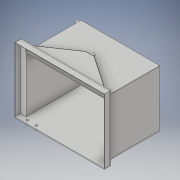
# Autodesk Inventor part: Tank2
Saved by Autodesk Inventor 2019 (Build 230136000, 136)
## iProperties
Created: 2020-03-11
Part Number: Tank2
Material: Generic
Document SubType Name: Modeling
Designer: Vijay
Density: 1 g/cm^3
Appearance: Default
Author: Vijay
Autodesk Inventor part; units mm, degrees
ref_plane "YZ Plane" through (0, 0, 0) normal (1, 0, 0) x (0, 1, 0)
ref_plane "XZ Plane" through (0, 0, 0) normal (0, 1, 0) x (-1, 0, 0)
ref_plane "XY Plane" through (0, 0, 0) normal (0, 0, 1) x (1, 0, 0)
sketch "Sketch1" plane through (0, 0, 0) normal (0, 0, 1) x (1, 0, 0)
  line L0 (-204, -167.1829) -> (204, -167.1829) construction
  line L1 (204, -167.1829) -> (204, 115) construction
  line L2 (204, 115) -> (-204, 115) construction
  line L3 (-204, 115) -> (-204, -167.1829) construction
  line L4 (-214, -177.1829) -> (214, -177.1829)
  line L5 (214, -177.1829) -> (214, 125)
  line L6 (214, 125) -> (-214, 125)
  line L7 (-214, 125) -> (-214, -177.1829)
  line L8 (-244, -177.1829) -> (244, -177.1829)
  line L9 (244, -177.1829) -> (244, 175)
  line L10 (244, 175) -> (-244, 175)
  line L11 (-244, 175) -> (-244, -177.1829)
  point P0 (0, 0)
  dimension "d0" = 10
  dimension "d1" = 30
  dimension "d2" = 30
  dimension "d3" = 50
  constraints: 24 end point, 6 parallel, 3 perpendicular, 2 horizontal, 5 other
  measures "d0" distance between parallel lines of L3 L7
  measures "d1" distance between parallel lines of L7 L11
  measures "d2" distance between parallel lines of L9 L5
  measures "d3" distance between parallel lines of L6 L10
extrude "Extrusion1" add sketch "Sketch1" along normal blind 5 contours L8 L11 L10 L9 L5 L6 L7
sketch "Sketch2" plane through (0, 0, 5) normal (0, 0, 1) x (1, 0, 0)
  line L0 (-214, -177.1829) -> (-214, 125) projected
  line L1 (-214, 125) -> (214, 125) projected
  line L2 (214, 125) -> (214, -177.1829) projected
  line L3 (214, -177.1829) -> (244, -177.1829) projected
  line L4 (244, -177.1829) -> (244, 175) projected
  line L5 (244, 175) -> (-244, 175) projected
  line L6 (-244, 175) -> (-244, -177.1829) projected
  line L7 (-244, -177.1829) -> (-214, -177.1829) projected
  line L8 (213.2, 124.2) -> (-213.2, 124.2)
  line L9 (-213.2, 124.2) -> (-213.2, -176.3829)
  line L10 (-244, -177.9829) -> (-244.8, -177.9829)
  line L11 (-244.8, -177.9829) -> (-244.8, 175.8)
  line L12 (-244.8, 175.8) -> (244.8, 175.8)
  line L13 (244.8, 175.8) -> (244.8, -177.9829)
  line L14 (244.8, -177.9829) -> (213.2, -177.9829)
  line L15 (214, 125) -> (214, -177.1829) projected
  line L16 (-244, -177.1829) -> (-214, -177.1829) projected
  line L17 (213.2, -177.1829) -> (-214, -177.1829)
  line L18 (213.2, -176.3829) -> (-213.2, -176.3829)
  line L19 (213.2, -177.1829) -> (214, -177.1829)
  line L20 (213.2, -177.9829) -> (213.2, -177.1829)
  line L21 (213.2, -176.3829) -> (213.2, 124.2)
  point P0 (0, 0)
  dimension "d6" = 0.8
  dimension "d7" = 0.8
  constraints: 24 end point, 2 horizontal, 1 perpendicular, 1 point on line, 3 other
  measures "d6" distance between parallel lines of L3 L14
  measures "d7" distance between parallel lines of L18 L17
extrude "Extrusion2" add sketch "Sketch2" against normal blind 300 contours L0 L1 L2 L19 L17
sketch "Sketch3" plane through (0, 0, 5) normal (0, 0, 1) x (1, 0, 0)
  line L0 (-213.2, -176.3829) -> (-213.2, 124.2) projected
  line L1 (-213.2, 124.2) -> (213.2, 124.2) projected
  line L2 (213.2, 124.2) -> (213.2, -176.3829) projected
  line L3 (213.2, -176.3829) -> (-213.2, -176.3829) projected
  line L4 (-244, -177.1829) -> (244, -177.1829) projected
  line L5 (244, -177.1829) -> (244, 175) projected
  line L6 (244, 175) -> (-244, 175) projected
  line L7 (-244, 175) -> (-244, -177.1829) projected
  line L8 (243.2, -176.3829) -> (-243.2, -176.3829)
  line L9 (-243.2, -176.3829) -> (-243.2, 174.2)
  line L10 (-243.2, 174.2) -> (243.2, 174.2)
  line L11 (243.2, 174.2) -> (243.2, -176.3829)
  point P0 (0, 0)
  dimension "d10" = 0.8
  constraints: 8 end point, 3 other
  measures "d10" distance between parallel lines of L4 L8
extrude "Extrusion3" add sketch "Sketch3" along normal blind 30
sketch "Sketch5" plane through (0, 0, -295) normal (0, 0, -1) x (-1, 0, 0)
  line L0 (213.2, 124.2) -> (213.2, -176.3829) projected
  line L1 (213.2, -176.3829) -> (-213.2, -176.3829) projected
  line L2 (-213.2, -176.3829) -> (-213.2, 124.2) projected
  line L3 (-213.2, 124.2) -> (213.2, 124.2) projected
  line L4 (-214, -177.1829) -> (214, -177.1829) projected
  line L5 (214, -177.1829) -> (214, 125) projected
  line L6 (214, 125) -> (-214, 125) projected
  line L7 (-214, 125) -> (-214, -177.1829) projected
  point P0 (0, 0)
extrude "Extrusion5" add sketch "Sketch5" along normal blind 0.8 contours L0 L1 L2 L3 | L7 L6 L5 L4
sketch "Sketch7" plane through (214, -177.1829, 0) normal (0, -1, 0) x (1, 0, 0)
  line L0 (0, 0) -> (30, 0) projected
  line L1 (30, 0) -> (30, 35) projected
  line L2 (-458, 35) -> (30, 35) projected
  line L3 (-458, 0) -> (-458, 35) projected
  line L4 (-458, 0) -> (-428, 0) projected
  line L5 (-428, 0) -> (-428, -295.8) projected
  line L6 (0, -295.8) -> (-428, -295.8) projected
  line L7 (0, 0) -> (0, -295.8) projected
  point P0 (-214, 0)
extrude "Extrusion7" add sketch "Sketch7" along normal blind 4.2
sketch "Sketch10" plane through (-214, 125, 0) normal (0, 1, 0) x (1, 0, 0)
  line L0 (428, 0) -> (0, 0) projected
  line L1 (428, 0) -> (428, 295.8) projected
  line L2 (0, 295.8) -> (428, 295.8) projected
  line L3 (0, 0) -> (0, 295.8) projected
  point P0 (214, 0)
extrude "Extrusion10" add sketch "Sketch10" along normal blind 4.2
sketch "Sketch12" plane through (0, 0, 5) normal (0, 0, 1) x (1, 0, 0)
  line L0 (214, 129.2) -> (-214, 129.2) projected
  line L1 (-214, 129.2) -> (214, 129.2)
  line L2 (214, 129.2) -> (214, 159.2)
  line L3 (214, 159.2) -> (-214, 159.2)
  line L4 (-214, 159.2) -> (-214, 129.2)
  point P0 (0, 0)
  dimension "d35" = 30
  constraints: 8 end point, 2 parallel, 1 horizontal, 1 perpendicular
  measures "d35" distance between parallel lines of L0 L3
extrude "Extrusion12" cut sketch "Sketch12" against normal through all
sketch "Sketch13" plane through (-214, 129.2, 0) normal (0, 1, 0) x (1, 0, 0)
  line L0 (428, -5) -> (428, 0) projected
  line L1 (0, -5) -> (0, 0) projected
  line L2 (214, -68.5291) -> (214, 358.2531) construction
  line L3 (428, 0) -> (235.9552, 130)
  line L4 (192.0448, 130) -> (0, 0)
  line L5 (-29.2, -5) -> (0.8, -5) projected
  line L6 (428, 0) -> (458, 0) projected
  line L7 (235.9552, 130) -> (192.0448, 130)
  line L8 (-0.8, 0.4245) -> (191.7995, 130.8)
  line L9 (191.7995, 130.8) -> (236.2005, 130.8)
  line L10 (236.2005, 130.8) -> (428.4485, 0.6625)
  line L11 (428.4485, 0.6625) -> (429.4271, 0)
  line L12 (-0.8, 0.4245) -> (-1.4271, 0)
  line L13 (429.4271, 0) -> (428, 0)
  line L14 (0, 0) -> (0, 295.8) projected
  line L15 (0, 0) -> (-1.4271, 0)
  point P0 (214, 0)
  point P1 (427.2, -5)
  dimension "d41" = 0.8
  constraints: 22 end point, 2 horizontal, 2 point on line, 1 perpendicular, 1 vertical, 2 other
  measures "d41" distance between parallel lines of L7 L9
extrude "Extrusion13" add sketch "Sketch13" along normal up to surface (30 mm away)
sketch "Sketch14" plane through (-22.2005, 159.2, -130.8) normal (0, 1, 0) x (1, 0, 0)
  line L0 (236.2005, -130.8) -> (44.1556, -0.8) projected
  line L1 (237.6276, -130.8) -> (236.2005, -130.8) projected
  line L2 (44.401, 0) -> (237.6276, -130.8) projected
  line L3 (0, 0) -> (44.401, 0) projected
  line L4 (-193.2266, -130.8) -> (0, 0) projected
  line L5 (-191.7995, -130.8) -> (-193.2266, -130.8) projected
  line L6 (0.2453, -0.8) -> (-191.7995, -130.8) projected
  line L7 (44.1556, -0.8) -> (0.2453, -0.8) projected
  line L8 (236.2005, -130.8) -> (44.1556, -0.8) projected
  line L9 (236.2005, -130.8) -> (-191.7995, -130.8) projected
  line L10 (236.2005, -130.8) -> (-191.7995, -130.8)
  point P0 (22.2005, -130.8)
  constraints: 2 end point, 2 point on line, 1 horizontal
extrude "Extrusion14" add sketch "Sketch14" along normal blind 0.8
sketch "Sketch15" plane through (-22.2005, 160, -130.8) normal (0, 1, 0) x (1, 0, 0)
  point P0 (22.2005, -130.8)
sketch "Sketch16" plane through (22.2005, 129.2, -130.8) normal (0, 0, -1) x (-1, 0, 0)
  circle A0 centre (22.2005, 18.5941) radius 7.5
  point P0 (22.2005, -129.2)
  dimension "d46" = 15
  constraints: 1 centre point
  measures "d46" diameter of A0
extrude "Extrusion15" cut sketch "Sketch16" against normal blind 0.8
sketch "Sketch17" plane through (22.2005, 129.2, -130.8) normal (0, 0, -1) x (-1, 0, 0)
  circle A0 centre (22.2005, 18.5941) radius 7.5 projected
  circle A1 centre (22.2005, 18.5941) radius 6.5
  point P0 (22.2005, -129.2)
  dimension "d49" = 1
  constraints: 1 centre point
  measures "d49" radial gap between concentric circles of A0 A1
extrude "Extrusion16" add sketch "Sketch17" along normal blind 20
sketch "Sketch18" plane through (214, -181.3829, 0) normal (0, -1, 0) x (1, 0, 0)
  circle A0 centre (-408, 17.5) radius 7.5
  circle A1 centre (-358, 17.5) radius 7.5
  line L0 (-458, 35) -> (-458, 0) projected
  point P0 (-214, 0)
  dimension "d52" = 15
  dimension "d53" = 15
  dimension "d54" = 50
  dimension "d55" = 50
  constraints: 2 centre point
  measures "d52" diameter of A0
  measures "d53" diameter of A1
  measures "d54" distance from line of L0 A0.centre
  measures "d55" distance of A0.centre A1.centre
extrude "Extrusion17" cut sketch "Sketch18" against normal blind 20
sketch "Sketch19" plane through (-243.2, -176.3829, 5) normal (0, 1, 0) x (1, 0, 0)
  circle A0 centre (99.2, -12.5) radius 7.5 projected
  circle A1 centre (49.2, -12.5) radius 7.5 projected
  circle A2 centre (99.2, -12.5) radius 6.5
  circle A3 centre (49.2, -12.5) radius 6.5
  point P0 (243.2, 5)
  dimension "d58" = 1
  dimension "d59" = 1
  constraints: 2 centre point
  measures "d58" radial gap between concentric circles of A0 A2
  measures "d59" radial gap between concentric circles of A1 A3
extrude "Extrusion18" add sketch "Sketch19" against normal blind 20
sketch "Sketch20" plane through (0, 147.7941, -130.8) normal (0, 0, 1) x (1, 0, 0)
  circle A0 centre (0, 0) radius 6.5 projected
  circle A1 centre (0, 0) radius 7.5 projected
  point P0 (0, -147.7941)
extrude "Extrusion19" add sketch "Sketch20" along normal up to surface (0.8 mm away)
sketch "Sketch21" plane through (-214, -181.3829, -295.8) normal (-1, 0, 0) x (0, 0, 1)
  line L0 (300.8, 305.5829) -> (0.8, 305.5829) projected
  line L1 (0.8, 305.5829) -> (0.8, 5) projected
  circle A0 centre (8.3, 298.0829) radius 7.5
  point P0 (295.8, 181.3829)
  dimension "d64" = 15
  constraints: 2 tangent, 1 centre point
  measures "d64" diameter of A0
extrude "Extrusion20" cut sketch "Sketch21" against normal blind 20 contours A0
sketch "Sketch22" plane through (-213.2, -176.3829, 5) normal (1, 0, 0) x (0, 0, -1)
  circle A0 centre (292.5, 293.0829) radius 7.5 projected
  circle A1 centre (292.5, 293.0829) radius 6.5
  point P0 (5, 176.3829)
  dimension "d67" = 1
  constraints: 1 centre point
  measures "d67" radial gap between concentric circles of A0 A1
extrude "Extrusion21" add sketch "Sketch22" against normal blind 20
body "Solid1"
